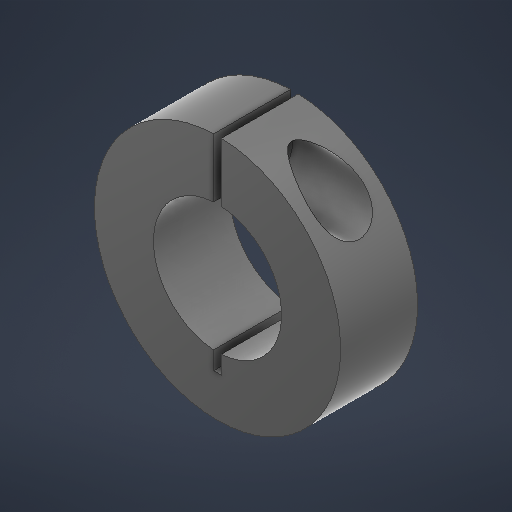
# Autodesk Inventor part: BagueSerrage
Saved by Autodesk Inventor 2026.2 (Build 302298010, 298A)
## iProperties
Created: 2026-04-20
Part Number: BagueSerrage
Material: Générique
Document SubType Name: Modeling
Designer: romai
Density: 1 g/cm^3
Appearance: Par défaut
Author: romai
Autodesk Inventor part; units mm, degrees
ref_plane "YZ Plane" through (0, 0, 0) normal (1, 0, 0) x (0, 1, 0)
ref_plane "XZ Plane" through (0, 0, 0) normal (0, 1, 0) x (-1, 0, 0)
sketch "Esquisse1" plane through (0, 0, 0) normal (0, 0, 1) x (1, 0, 0)
  circle A0 centre (0, 0) radius 12.5
  circle A1 centre (0, 0) radius 24
  dimension "d0" = 25
  dimension "d1" = 48
  constraints: 2 centre point, 2 coincident
  measures "d0" diameter of A0
  measures "d1" diameter of A1
extrude "Extrusion1" add sketch "Esquisse1" along normal mid plane 15
sketch "Esquisse2" plane through (0, 0, 7.5) normal (0, 0, 1) x (1, 0, 0)
  line L0 (-0.75, 24) -> (0.75, 24)
  line L1 (0.75, 24) -> (0.75, -16)
  line L2 (0.75, -16) -> (-0.75, -16)
  line L3 (-0.75, -16) -> (-0.75, 24)
  line L4 (-0.75, 24) -> (0.75, -16) construction
  line L5 (0.75, 24) -> (-0.75, -16) construction
  circle A0 centre (0, 0) radius 24 projected
  point P0 (0, 4)
  dimension "d4" = 1.5
  dimension "d5" = 40
  constraints: 12 end point, 2 midpoint, 2 parallel, 1 horizontal, 1 perpendicular, 1 tangent
  measures "d4" distance of L1.end L2.end
  measures "d5" distance of L0.end L1.end
extrude "Extrusion2" cut sketch "Esquisse2" against normal through all contours L0 A0 L3 | L0 L1 A0 | A0 L1 L2 L3 picked at (0, -2.6667)
ref_plane "Plan de construction1" through (4.25, 12.4775, 7.5) normal (1, 0, 0) x (0, 0, -1)
sketch "Esquisse3" plane through (4.25, 12.4775, 7.5) normal (1, 0, 0) x (0, 0, -1)
  line L0 (0, 11.5108) -> (15, 11.5108) projected
  line L1 (0, 0) -> (0, 11.5108) projected
  line L2 (15, 0) -> (0, 0) projected
  line L3 (15, 11.5108) -> (15, 0) projected
  point P0 (7.5, -12.4775)
  point P1 (7.4264, 5.4735)
hole "Perçage1" at (4.25, 17.951, 0.0736) direction (-1, 0, 0) diameter 4.134 depth 14 counterbore diameter 10 counterbore depth 2 thread size "M5x0.8" class "6H" standard "ISO Metric profile"
sketch "Esquisse4" plane through (4.25, 12.4775, 7.5) normal (1, 0, 0) x (0, 0, -1)
  circle A0 centre (7.4264, 5.4735) radius 5 projected
  point P0 (7.5, -12.4775)
extrude "Extrusion3" cut sketch "Esquisse4" along normal through all
